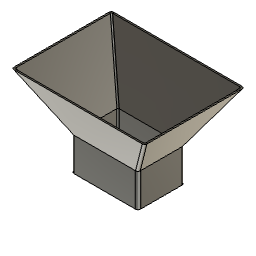
05 (Autodesk Fusion 360 design; units mm, degrees)
Autodesk Fusion 360 part; units mm, degrees
sketch "Sketch1" plane through (0, 0, 0) normal (0, 0, 1) x (1, 0, 0)
  line L0 (0, 0) -> (100, 0)
  line L1 (100, 0) -> (100, 70)
  line L2 (100, 70) -> (0, 70)
  line L3 (0, 70) -> (0, 0)
  dimension "d1" = 100
  dimension "d2" = 70
  constraint horizontal L0
  constraint vertical L1
  constraint horizontal L2
  constraint vertical L3
  constraint coincident L0.start L3.end
  measures "d1" distance of L0.start L0.end
  measures "d2" distance of L0.start L2.end
ref_plane "WorkPlane1" through (50, 35, 80) normal (0, 0, 1) x (1, 0, 0)
sketch "Sketch2" plane through (50, 35, 80) normal (0, 0, 1) x (1, 0, 0)
  line L0 (100, 75) -> (-100, 75)
  line L1 (-100, 75) -> (-100, -75)
  line L2 (-100, -75) -> (100, -75)
  line L3 (100, -75) -> (100, 75)
  line L4 (100, 75) -> (-100, -75) construction
  line L5 (-100, 75) -> (100, -75) construction
  dimension "d4" = 200
  dimension "d5" = 150
  constraint horizontal L0
  constraint perpendicular L0 L1
  constraint parallel L0 L2
  constraint parallel L1 L3
  constraint coincident L4 origin
  constraint coincident L5 origin
  measures "d4" distance of L1.end L2.end
  measures "d5" distance of L0.end L1.end
loft "Loft1" add profiles "Sketch1", "Sketch2" section 1 section 2
extrude "Extrude1" add 1 faces at (33.3333, 23.3333, 0) along direction (0, 0, -1) blind 50
fillet "Fillet1" radius 4 8 edges at (-25, -20, 40) (125, -20, 40) (125, 90, 40) (-25, 90, 40) (0, 70, -25) (0, 0, -25) (100, 0, -25) (100, 70, -25)
shell "Shell1" thickness 2 removed faces 2 at (17.8663, 10, 80) at (65.3333, 46.6667, -50)
